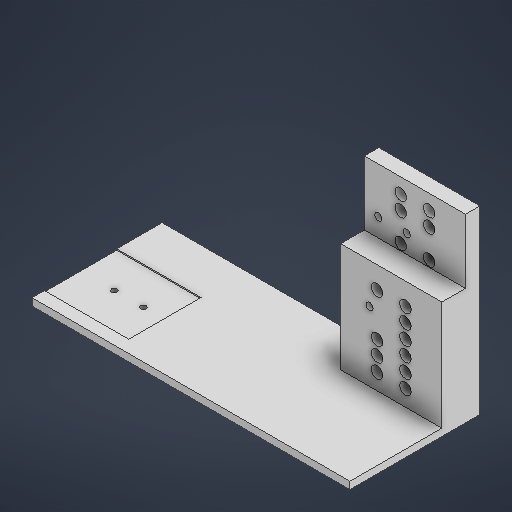
# Autodesk Inventor part: Baseplate as 1 V3
Saved by Autodesk Inventor 2026 (Build 300175000, 175)
## iProperties
Created: 2025-12-17
Part Number: Baseplate as 1 V3
Material: Generic
Document SubType Name: Modeling
Designer: FiolkaLab
Density: 1 g/cm^3
Appearance: Default
Author: FiolkaLab
Autodesk Inventor part; units mm, degrees
ref_plane "YZ Plane" through (0, 0, 0) normal (1, 0, 0) x (0, 1, 0)
ref_plane "XZ Plane" through (0, 0, 0) normal (0, 1, 0) x (-1, 0, 0)
ref_plane "XY Plane" through (0, 0, 0) normal (0, 0, 1) x (1, 0, 0)
sketch "Sketch1" plane through (0, 0, 0) normal (0, 0, 1) x (1, 0, 0)
  line L0 (44.45, 76.2) -> (-44.45, 76.2)
  line L1 (-44.45, 76.2) -> (-44.45, -76.2)
  line L2 (-44.45, -76.2) -> (44.45, -76.2)
  line L3 (44.45, -76.2) -> (44.45, 76.2)
  line L4 (44.45, 76.2) -> (-44.45, -76.2) construction
  line L5 (-44.45, 76.2) -> (44.45, -76.2) construction
  point P0 (0, 0)
  dimension "d0" = 152.4
  dimension "d1" = 88.9
  constraints: 12 end point, 2 midpoint, 2 parallel, 1 horizontal, 1 perpendicular
  measures "d0" distance of L2.end L0.start
  measures "d1" distance of L0.start L0.end
extrude "Extrusion1" add sketch "Sketch1" along normal blind 12.7
sketch "Sketch2" plane through (0, 0, 12.7) normal (0, 0, 1) x (1, 0, 0)
  line L0 (-44.45, 76.2) -> (-44.45, -76.2) projected
  line L1 (44.45, -76.2) -> (44.45, 76.2) projected
  line L2 (-44.45, -76.2) -> (44.45, -76.2)
  line L3 (44.45, -76.2) -> (44.45, 19.812)
  line L4 (44.45, 19.812) -> (-44.45, 19.812)
  line L5 (-44.45, 19.812) -> (-44.45, -76.2)
  point P0 (0, 0)
  dimension "d4" = 96.012
  constraints: 8 end point, 2 parallel, 1 horizontal, 1 perpendicular, 1 point on line
  measures "d4" distance between parallel lines of L2 L4
extrude "Extrusion2" add sketch "Sketch2" along normal blind 20.828
sketch "Sketch3" plane through (0, 0, 0) normal (0, 0, -1) x (-1, 0, 0)
  line L0 (-44.45, -76.2) -> (-44.45, 76.2) projected
  line L1 (44.45, -76.2) -> (-44.45, -76.2) projected
  point P0 (0, 0)
  point P1 (19.05, -15.24)
  dimension "d14" = 63.5
  dimension "d15" = 60.96
  measures "d14" distance from line of L0 point (19.05, -15.24)
  measures "d15" distance from line of L1 point (19.05, -15.24)
hole "Hole1" at (-19.05, -15.24, 0) direction (0, 0, 1) diameter 6.35 end through all counterbore diameter 10.16 counterbore depth 7.62
sketch "Sketch4" plane through (0, 0, 0) normal (0, 0, -1) x (-1, 0, 0)
  line L0 (44.45, -76.2) -> (-44.45, -76.2) projected
  line L1 (-44.45, -76.2) -> (-44.45, 76.2) projected
  point P0 (0, 0)
  point P1 (32.1564, 35.937)
  point P2 (44.45, 19.812)
  dimension "d24" = 76.6064
  dimension "d155" = 16.125
  measures "d24" distance from line of L1 point (32.156, 35.937)
  measures "d155" vertical distance of point (44.45, 19.812) point (32.156, 35.937)
hole "Hole2" at (-32.1564, 35.937, 0) direction (0, 0, 1) diameter 6.35 end through all counterbore diameter 10.16 counterbore depth 7.62
pattern_linear "Rectangular Pattern1" count 2 spacing 25 along (1, 0, 0) of "Hole2"
sketch "Sketch5" plane through (0, 0, 12.7) normal (0, 0, 1) x (1, 0, 0)
  line L0 (-44.45, 76.2) -> (-44.45, 19.812) projected
  line L1 (44.45, 76.2) -> (-44.45, 76.2) projected
  point P0 (0, 0)
  point P1 (-12.5, 62.9666)
  dimension "d35" = 31.95
  dimension "d36" = 13.2334
  measures "d35" distance from line of L0 point (-12.5, 62.967)
  measures "d36" distance from line of L1 point (-12.5, 62.967)
hole "Hole3" at (-12.5, 62.9666, 12.7) direction (0, 0, -1) diameter 6.35 end through all counterbore diameter 10.16 counterbore depth 7.62
pattern_linear "Rectangular Pattern2" count 2 spacing 25 along (1, 0, 0) count 2 spacing 12.5 along (0, -1, 0) of "Hole3"
sketch "Sketch6" plane through (0, 0, 12.7) normal (0, 0, 1) x (1, 0, 0)
  circle A0 centre (-12.5, 50.4666) radius 5.08 projected
  line L0 (-44.45, 76.2) -> (-44.45, 19.812) projected
  point P0 (0, 0)
  point P1 (-12.5, 25.4666)
  dimension "d50" = 25
  dimension "d51" = 31.95
  measures "d50" distance of A0.centre point (-12.5, 25.467)
  measures "d51" distance from line of L0 point (-12.5, 25.467)
hole "Hole4" at (-12.5, 25.4666, 12.7) direction (0, 0, -1) diameter 6.35 end through all counterbore diameter 10.16 counterbore depth 7.62
pattern_linear "Rectangular Pattern3" count 2 spacing 25 along (1, 0, 0) of "Hole4"
sketch "Sketch7" plane through (0, 0, 33.528) normal (0, 0, 1) x (1, 0, 0)
  line L0 (-44.45, 19.812) -> (-44.45, -76.2) projected
  circle A0 centre (-12.5, 25.4666) radius 3.175 projected
  point P0 (0, 0)
  point P1 (-12.5, 0.4666)
  dimension "d62" = 31.95
  dimension "d63" = 25
  measures "d62" distance from line of L0 point (-12.5, 0.467)
  measures "d63" distance of A0.centre point (-12.5, 0.467)
hole "Hole5" at (-12.5, 0.4666, 33.528) direction (0, 0, -1) diameter 6.35 end through all counterbore diameter 10.16 counterbore depth 7.62
pattern_linear "Rectangular Pattern4" count 2 spacing 25 along (1, 0, 0) of "Hole5"
sketch "Sketch8" plane through (0, 0, 33.528) normal (0, 0, 1) x (1, 0, 0)
  line L0 (-44.45, 19.812) -> (-44.45, -76.2) projected
  circle A0 centre (-12.5, 0.4666) radius 5.08 projected
  point P0 (0, 0)
  point P1 (-12.5, -37.0334)
  dimension "d74" = 31.95
  dimension "d75" = 37.5
  measures "d74" distance from line of L0 point (-12.5, -37.033)
  measures "d75" distance of A0.centre point (-12.5, -37.033)
hole "Hole6" at (-12.5, -37.0334, 33.528) direction (0, 0, -1) diameter 6.35 end through all counterbore diameter 10.16 counterbore depth 7.62
pattern_linear "Rectangular Pattern5" count 2 spacing 25 along (1, 0, 0) count 3 spacing 12.5 along (0, -1, 0) of "Hole6"
sketch "Sketch9" plane through (0, 0, 33.528) normal (0, 0, 1) x (1, 0, 0)
  line L0 (44.45, -76.2) -> (44.45, 19.812) projected
  circle A0 centre (12.5, 0.4666) radius 5.08 projected
  point P0 (0, 0)
  point P1 (12.5, -12.0334)
  dimension "d89" = 31.95
  dimension "d90" = 12.5
  measures "d89" distance from line of L0 point (12.5, -12.033)
  measures "d90" distance of A0.centre point (12.5, -12.033)
hole "Hole7" at (12.5, -12.0334, 33.528) direction (0, 0, -1) diameter 6.35 end through all counterbore diameter 10.16 counterbore depth 7.62
pattern_linear "Rectangular Pattern6" count 2 spacing 12.5 along (0, -1, 0) of "Hole7"
sketch "Sketch13" plane through (-44.45, -76.2, 0) normal (0, -1, 0) x (1, 0, 0)
  line L0 (88.9, 0) -> (0, 0) projected
  line L1 (88.9, 0) -> (-190.5, 0)
  line L2 (-190.5, 0) -> (-190.5, 114.3)
  line L3 (-190.5, 114.3) -> (88.9, 114.3)
  line L4 (88.9, 114.3) -> (88.9, 0)
  point P0 (44.45, 0)
  dimension "d133" = 279.4
  dimension "d134" = 114.3
  constraints: 8 end point, 2 parallel, 1 horizontal, 1 perpendicular
  measures "d133" distance of L2.end L3.end
  measures "d134" distance of L1.end L2.end
extrude "Extrusion3" add sketch "Sketch13" along normal blind 6.35
sketch "Sketch14" plane through (-44.45, -76.2, 0) normal (0, 1, 0) x (1, 0, 0)
  line L0 (88.9, 0) -> (88.9, -114.3) projected
  line L1 (-190.5, 0) -> (0, 0) projected
  point P0 (44.45, 0)
  point P1 (-135.4328, -71.628)
  dimension "d144" = 224.3328
  dimension "d145" = 71.628
  measures "d144" distance from line of L0 point (-135.433, -71.628)
  measures "d145" distance from line of L1 point (-135.433, -71.628)
hole "Hole11" at (-179.8828, -76.2, 71.628) direction (0, -1, 0) diameter 4.9784 end through all thread size "1/4-20 UNC" class "2B" standard "ANSI Unified Screw Threads"
pattern_linear "Rectangular Pattern10" count 2 spacing 25.4 along (-1, 0, 0) of "Hole11"
sketch "Sketch15" plane through (-44.45, -76.2, 0) normal (0, 1, 0) x (1, 0, 0)
  line L0 (-116.3828, -39.878) -> (-192.5828, -39.878)
  line L1 (-192.5828, -39.878) -> (-192.5828, -103.378)
  line L2 (-192.5828, -103.378) -> (-116.3828, -103.378)
  line L3 (-116.3828, -103.378) -> (-116.3828, -39.878)
  circle A0 centre (-135.4328, -71.628) radius 2.4892 projected
  point P0 (44.45, 0)
  dimension "d149" = 63.5
  dimension "d150" = 76.2
  dimension "d151" = 19.05
  dimension "d152" = 31.75
  constraints: 8 end point, 2 parallel, 1 horizontal, 1 perpendicular
  measures "d149" distance of L2.end L0.start
  measures "d150" distance of L1.end L2.end
  measures "d151" distance from line of L3 A0.centre
  measures "d152" distance from line of L2 A0.centre
extrude "Extrusion4" cut sketch "Sketch15" against normal blind 1.0414
body "Solid1"
